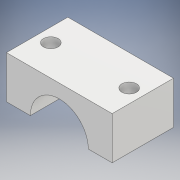
# Autodesk Inventor part: Colimador superior
Saved by Autodesk Inventor 2019.4 (Build 234330000, 330)
## iProperties
Created: 2018-03-06
Part Number: Colimador superior
Material: Generic
Document SubType Name: Modeling
Designer: Hogar
Density: 1 g/cm^3
Appearance: White
Author: Hogar
Autodesk Inventor part; units mm, degrees
ref_plane "YZ Plane" through (0, 0, 0) normal (1, 0, 0) x (0, 1, 0)
ref_plane "XZ Plane" through (0, 0, 0) normal (0, 1, 0) x (-1, 0, 0)
ref_plane "XY Plane" through (0, 0, 0) normal (0, 0, 1) x (1, 0, 0)
sketch "Sketch1" plane through (0, 0, 0) normal (0, 0, 1) x (1, 0, 0)
  line L0 (-15.5, -9) -> (15.5, -9)
  line L1 (15.5, -9) -> (15.5, 9)
  line L2 (15.5, 9) -> (-15.5, 9)
  line L3 (-15.5, 9) -> (-15.5, -9)
  line L4 (-15.5, -9) -> (15.5, 9) construction
  line L5 (15.5, -9) -> (-15.5, 9) construction
  point P0 (0, 0)
  dimension "d0" = 31
  dimension "d1" = 18
  constraints: 12 end point, 2 midpoint, 2 parallel, 1 horizontal, 1 perpendicular
  measures "d0" distance of L2.end L1.end
  measures "d1" distance of L1.end L0.end
extrude "Extrusion1" add sketch "Sketch1" along normal blind 12.5
sketch "Sketch8" plane through (-15.5, -9, 0) normal (0, -1, 0) x (1, 0, 0)
  circle A0 centre (15.5, 0) radius 7.5
  dimension "d57" = 15
  constraints: 1 centre point, 1 coincident
  measures "d57" diameter of A0
extrude "Extrusion8" cut sketch "Sketch8" against normal through all
sketch "Sketch9" plane through (0, 0, 12.5) normal (0, 0, 1) x (1, 0, 0)
  line L0 (-15.5, -9) -> (15.5, -9) projected
  point P0 (0, 0)
  point P1 (-11.5, 0)
  point P2 (11.5, 0)
  dimension "d68" = 11.5
  dimension "d69" = 11.5
  dimension "d70" = 9
  dimension "d71" = 9
  measures "d68" distance of point (0, 0) point (-11.5, 0)
  measures "d69" distance of point (11.5, 0) point (0, 0)
  measures "d70" distance from line of L0 point (-11.5, 0)
  measures "d71" distance from line of L0 point (11.5, 0)
hole "Hole1" at (-11.5, 0, 12.5) at (11.5, 0, 12.5) direction (0, 0, -1) diameter 4.3 end through all clearance for "Flat Head Machine Screw" size "M4" standard "Ansi Metric M Profile"
sketch "Sketch10" plane through (-15.5, -9, 12.5) normal (0, -1, 0) x (1, 0, 0)
  arc A0 (23, -12.5) -> (8, -12.5) centre (15.5, -12.5) ccw projected
  circle A1 centre (15.5, -12.5) radius 8.5
  dimension "d79" = 17
  constraints: 1 centre point, 1 coincident
  measures "d79" diameter of A1
extrude "Extrusion10" cut sketch "Sketch10" against normal blind 9
equation "\"d69\" = d68"
equation "\"d71\" = d70"
body "Solid1"
